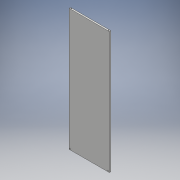
# Autodesk Inventor part: sideplate part 1
Saved by Autodesk Inventor 2018 (Build 220112000, 112)
## iProperties
Created: 2018-06-15
Part Number: sideplate part 1
Material: Generic
Document SubType Name: Modeling
Designer: John Viljoen
Density: 1 g/cm^3
Appearance: Default
Author: John Viljoen
Autodesk Inventor part; units mm, degrees
ref_plane "YZ Plane" through (0, 0, 0) normal (1, 0, 0) x (0, 1, 0)
ref_plane "XZ Plane" through (0, 0, 0) normal (0, 1, 0) x (-1, 0, 0)
ref_plane "XY Plane" through (0, 0, 0) normal (0, 0, 1) x (1, 0, 0)
sketch "Sketch1" plane through (0, 0, 0) normal (0, 0, 1) x (1, 0, 0)
  line L0 (0, 0) -> (109.5, 0)
  line L1 (109.5, 0) -> (109.5, 4)
  line L2 (109.5, 4) -> (0, 4)
  line L3 (0, 4) -> (0, 0)
  dimension "d0" = 109.5
  dimension "d1" = 4
  constraints: 8 end point, 2 parallel, 1 horizontal, 1 perpendicular
  measures "d0" distance of L2.end L1.end
  measures "d1" distance of L1.end L0.end
extrude "Extrusion1" add sketch "Sketch1" along normal blind 332.175
sketch "Sketch2" plane through (0, 0, 0) normal (0, -1, 0) x (1, 0, 0)
  line L0 (0, 0) -> (109.5, 0) projected
  line L1 (0, 0) -> (3.175, 0) construction
  line L2 (3.175, 0) -> (3.175, 3.175) construction
  circle A0 centre (3.175, 3.175) radius 1.25
  line L3 (109.5, 0) -> (106.325, 0) construction
  line L4 (106.325, 0) -> (106.325, 3.175) construction
  circle A1 centre (106.325, 3.175) radius 1.25
  dimension "d4" = 3.175
  dimension "d5" = 3.175
  dimension "d6" = 2.5
  dimension "d7" = 3.175
  dimension "d8" = 3.175
  dimension "d9" = 2.5
  constraints: 8 end point, 2 centre point, 2 coincident, 2 perpendicular, 2 point on line
  measures "d4" distance of L0.start L1.end
  measures "d5" distance of L1.end L2.end
  measures "d6" diameter of A0
  measures "d7" distance of L0.end L3.end
  measures "d8" distance of L3.end L4.end
  measures "d9" diameter of A1
extrude "Extrusion2" cut sketch "Sketch2" against normal blind 10
sketch "Sketch3" plane through (0, 0, 332.175) normal (0, 0, 1) x (1, 0, 0)
  line L0 (0, 0) -> (109.5, 0) projected
  line L1 (109.5, 0) -> (109.5, 4) projected
  line L2 (0, 0) -> (4, 0) construction
  line L3 (4, 0) -> (4, 2) construction
  circle A0 centre (4, 2) radius 1
  line L4 (109.5, 2) -> (105.5, 2) construction
  circle A1 centre (105.5, 2) radius 1
  dimension "d12" = 4
  dimension "d13" = 2
  dimension "d14" = 2
  dimension "d15" = 4
  dimension "d16" = 2
  constraints: 6 end point, 2 centre point, 2 coincident, 1 horizontal, 1 midpoint, 1 perpendicular, 1 point on line
  measures "d12" distance of L0.start L2.end
  measures "d13" distance of L2.end L3.end
  measures "d14" diameter of A0
  measures "d15" distance of L4.start L4.end
  measures "d16" diameter of A1
extrude "Extrusion3" cut sketch "Sketch3" against normal blind 10
body "Solid1"
